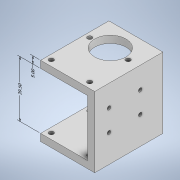
# Autodesk Inventor part: サーボモータ固定２軸
Saved by Autodesk Inventor 2022 (Build 260153000, 153)
## iProperties
Created: 2022-11-23
Part Number: サーボモータ固定２軸
Material: 一般
Document SubType Name: Modeling
Designer: tdn82
Density: 1 g/cm^3
Appearance: 既定
Author: tdn82
Autodesk Inventor part; units mm, degrees
ref_plane "YZ Plane" through (0, 0, 0) normal (1, 0, 0) x (0, 1, 0)
ref_plane "XZ Plane" through (0, 0, 0) normal (0, 1, 0) x (-1, 0, 0)
ref_plane "XY Plane" through (0, 0, 0) normal (0, 0, 1) x (1, 0, 0)
sketch "スケッチ1" plane through (0, 0, 0) normal (0, 1, 0) x (-1, 0, 0)
  line L0 (0, 0) -> (-38, 0)
  line L1 (-38, 0) -> (-38, -48)
  line L2 (-38, -48) -> (0, -48)
  line L3 (0, -48) -> (0, 0)
  dimension "d0" = 48
  dimension "d1" = 38
  constraints: 8 end point, 2 parallel, 1 horizontal, 1 perpendicular
  measures "d0" distance of L0.end L1.end
  measures "d1" distance of L1.end L2.end
extrude "押し出し1" add sketch "スケッチ1" along normal blind 49.5
sketch "スケッチ2" plane through (38, 0, -48) normal (0, 0, -1) x (-1, 0, 0)
  line L0 (5, 44.5) -> (59.072, 44.5)
  line L1 (59.072, 44.5) -> (59.072, 5)
  line L2 (59.072, 5) -> (5, 5)
  line L3 (5, 5) -> (5, 44.5)
  line L4 (0, 49.5) -> (38, 49.5) projected
  line L5 (0, 0) -> (38, 0) projected
  line L6 (0, 0) -> (0, 49.5) projected
  dimension "d4" = 39.5
  dimension "d6" = 5
  dimension "d7" = 5
  constraints: 8 end point, 2 parallel, 1 horizontal, 1 perpendicular
  measures "d4" distance of L2.end L0.start
  measures "d6" distance between parallel lines of L2 L5
  measures "d7" distance between parallel lines of L6 L3
extrude "押し出し2" cut sketch "スケッチ2" against normal blind 100
sketch "スケッチ3" plane through (0, 49.5, 0) normal (0, 1, 0) x (1, 0, 0)
  line L0 (38, 48) -> (0, 48) projected
  line L1 (38, 0) -> (38, 48) projected
  point P0 (0, 0)
  point P1 (17, 32)
  dimension "d10" = 16
  dimension "d11" = 21
  measures "d10" distance from line of L0 point (17, 32)
  measures "d11" distance from line of L1 point (17, 32)
hole "穴1" at (17, 49.5, -32) direction (0, -1, 0) diameter 22 end through all
sketch "スケッチ4" plane through (0, 49.5, 0) normal (0, 1, 0) x (1, 0, 0)
  line L0 (0, 0) -> (38, 0) projected
  line L1 (38, 0) -> (38, 48) projected
  point P0 (30.5, 4)
  point P1 (30.5, 31)
  point P2 (3.5, 4)
  point P3 (3.5, 31)
  point P4 (3.5, 4)
  dimension "d19" = 4
  dimension "d20" = 7.5
  dimension "d23" = 27
  dimension "d26" = 27
  constraints: 1 coincident, 1 horizontal, 1 vertical, 3 other
  measures "d19" distance from line of L0 point (30.5, 4)
  measures "d20" distance from line of L1 point (30.5, 4)
  measures "d23" distance of point (30.5, 4) point (30.5, 31)
  measures "d26" distance of point (30.5, 4) point (3.5, 4)
hole "穴2" at (30.5, 49.5, -4) at (30.5, 49.5, -31) at (3.5, 49.5, -31) at (3.5, 49.5, -4) direction (0, -1, 0) diameter 3.2 end through all
sketch "スケッチ6" plane through (38, 0, 0) normal (1, 0, 0) x (0, 0, -1)
  line L0 (0, 49.5) -> (48, 49.5) projected
  line L1 (0, 0) -> (0, 49.5) projected
  point P0 (10, 34.5)
  point P1 (32, 34.5)
  point P2 (10, 19.5)
  point P3 (32, 19.5)
  dimension "d45" = 15
  dimension "d46" = 10
  dimension "d49" = 22
  dimension "d52" = 15
  constraints: 1 horizontal, 1 vertical, 3 other
  measures "d45" distance from line of point (10, 34.5) L0
  measures "d46" distance from line of L1 point (10, 34.5)
  measures "d49" distance of point (10, 34.5) point (32, 34.5)
  measures "d52" distance of point (10, 34.5) point (10, 19.5)
hole "穴4" at (38, 34.5, -10) at (38, 34.5, -32) at (38, 19.5, -10) at (38, 19.5, -32) direction (-1, 0, 0) diameter 2.5 end through all
